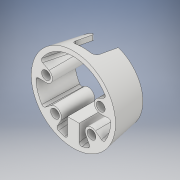
# Autodesk Inventor part: baseBottom
Saved by Autodesk Inventor 2018 (Build 220112000, 112)
## iProperties
Created: 2017-04-10
Part Number: baseBottom
Material: ABS Plastic
Document SubType Name: Modeling
Designer: dkt01
Density: 1.06 g/cm^3
Appearance: Smooth - White
Author: dkt01
Autodesk Inventor part; units mm, degrees
ref_plane "YZ Plane" through (0, 0, 0) normal (1, 0, 0) x (0, 1, 0)
ref_plane "XZ Plane" through (0, 0, 0) normal (0, 1, 0) x (-1, 0, 0)
sketch "Sketch1" plane through (0, 0, 0) normal (0, 0, 1) x (1, 0, 0)
  circle A0 centre (0, 0) radius 30.643
  circle A1 centre (0, 0) radius 26.581
  line L0 (0, 0) -> (0, 34.214349)
  line L1 (10, 28.965384) -> (10, 24.628227)
  line L2 (-24, 19.052387) -> (-24, 11.425829)
  dimension "d51" = 53.162
  dimension "d53" = 10
  dimension "d54" = 24
  dimension "d55" = 4.062
  constraints: 6 end point, 4 point on circle, 3 vertical, 2 centre point, 2 coincident
  measures "d51" diameter of A1
  measures "d53" distance between parallel lines of L0 L1
  measures "d54" distance between parallel lines of L2 L0
  measures "d55" radial gap between concentric circles of A0 A1
extrude "Extrusion1" add sketch "Sketch1" along normal blind 30 draft 10
shell "Shell1" thickness 4 removed faces 2 at (10.151889, -4.096582, 30) at (-7.737173, 3.588786, 0)
sketch "Sketch2" plane through (0, 0, 0) normal (0, 0, -1) x (-1, 0, 0)
  line L0 (0, 0) -> (0, 42.956518)
  line L1 (-10, 5.652174) -> (10, 5.652174)
  line L2 (10, 5.652174) -> (10, 52.710838)
  line L3 (10, 52.710838) -> (-10, 52.710838)
  line L4 (-10, 52.710838) -> (-10, 5.652174)
  dimension "d3" = 10
  dimension "d4" = 10
  constraints: 10 end point, 2 parallel, 1 horizontal, 1 perpendicular, 1 vertical
  measures "d3" distance between parallel lines of L0 L4
  measures "d4" distance between parallel lines of L2 L0
extrude "Extrusion2" cut sketch "Sketch2" against normal blind 22
ref_plane "Work Plane1" through (0, 0, 1.7) normal (0, 0, -1) x (-1, 0, 0)
sketch "Sketch3" plane through (0, 0, 1.7) normal (0, 0, -1) x (-1, 0, 0)
  arc A0 (-10, 24.628544) -> (10, 24.628544) centre (0, 0) ccw
  circle A1 centre (-23.304766, 6.454224) radius 2
  circle A2 centre (-15.445766, -18.129473) radius 2
  circle A3 centre (15.640493, -18.228751) radius 2
  circle A4 centre (23.319503, 6.396996) radius 2
  circle A5 centre (-23.304766, 6.454224) radius 3.75
  circle A6 centre (-15.445766, -18.129473) radius 3.75
  circle A7 centre (15.640493, -18.228751) radius 3.75
  circle A8 centre (23.319503, 6.396996) radius 3.75
  circle A9 centre (-23.304766, 6.454224) radius 5.5
  circle A10 centre (-15.445766, -18.129473) radius 5.5
  circle A11 centre (15.640493, -18.228751) radius 5.5
  circle A12 centre (23.319503, 6.396996) radius 5.5
  line L0 (-20.945766, 0) -> (17.819503, 0)
  line L1 (-23.304766, 6.454224) -> (0, 0)
  line L2 (0, 0) -> (23.319503, 6.396996)
  line L3 (15.640493, -18.228751) -> (0, 0)
  line L4 (0, 0) -> (-15.445766, -18.129473)
  dimension "d19" = 4
  dimension "d20" = 4
  dimension "d21" = 4
  dimension "d22" = 4
  dimension "d23" = 7.5
  dimension "d24" = 7.5
  dimension "d25" = 7.5
  dimension "d26" = 7.5
  dimension "d29" = 11
  dimension "d30" = 11
  dimension "d31" = 11
  dimension "d32" = 11
  dimension "d56" = 15.34
  dimension "d57" = 15.48
  dimension "d58" = 49.57
  dimension "d59" = 49.37
  dimension "d60" = 24.181
  dimension "d61" = 24.182
  dimension "d62" = 23.817
  dimension "d63" = 24.019
  constraints: 12 centre point, 12 coincident, 10 end point, 1 horizontal
  measures "d19" diameter of A1
  measures "d20" diameter of A2
  measures "d21" diameter of A3
  measures "d22" diameter of A4
  measures "d23" diameter of A5
  measures "d24" diameter of A6
  measures "d25" diameter of A7
  measures "d26" diameter of A8
  measures "d29" diameter of A9
  measures "d30" diameter of A10
  measures "d31" diameter of A12
  measures "d32" diameter of A11
  measures "d56" angle of L0 L2
  measures "d57" angle of L0 L1
  measures "d58" angle of L4 L0
  measures "d59" angle of L3 L0
  measures "d60" distance of L1.end L2.end
  measures "d61" distance of L1.start L1.end
  measures "d62" distance of L1.end L4.end
  measures "d63" distance of L3.start L1.end
sketch "Sketch4" plane through (0, 0, 30) normal (0, 0, 1) x (1, 0, 0)
  line L0 (5, -15) -> (-5, -15)
  line L1 (-5, -15) -> (-5, -35.527022)
  line L2 (-5, -35.527022) -> (5, -35.527022)
  line L3 (5, -35.527022) -> (5, -15)
  line L4 (0, 0) -> (0, -18.124685)
  dimension "d11" = 5
  dimension "d12" = 5
  dimension "d13" = 15
  constraints: 10 end point, 2 parallel, 1 horizontal, 1 perpendicular, 1 vertical
  measures "d11" distance between parallel lines of L4 L3
  measures "d12" distance between parallel lines of L1 L4
  measures "d13" distance from line of L4.start L0
extrude "Extrusion3" add sketch "Sketch4" against normal up to surface (28.3 mm away) from surface at 0
fillet "Fillet1" radius 2 2 edges at (-5, -28.8365, 15.2299) (5, -28.8365, 15.2299)
sketch "Sketch5" plane through (0, 0, 1.7) normal (0, 0, -1) x (-1, 0, 0)
  arc A0 (-5, -30.536112) -> (5, -30.536112) centre (0, 0) ccw
  line L0 (-5, -35.527022) -> (-5, -30.536112)
  line L1 (5, -35.527022) -> (-5, -35.527022)
  line L2 (5, -30.536112) -> (5, -35.527022)
extrude "Extrusion4" cut sketch "Sketch5" against normal up to surface round surface about axis through (0, 0, 0) along (0, 0, 1) radius 30.643 half angle 10 far side no
extrude "Extrusion5" cut sketch "Sketch3" against normal up to surface (30 mm away) from surface at 1.7 contours A5 A0 | A0 A5 | A6 A0 | A0 A6 | A8 A0 | A7 A0 | A0 A7 | A8 A0 | A1 | A2 | A3 | A4
ref_plane "Work Plane2" through (0, 0, 4.7) normal (0, 0, -1) x (-1, 0, 0)
sketch "Sketch6" plane through (0, 0, 4.7) normal (0, 0, -1) x (-1, 0, 0)
  circle A0 centre (15.640493, -18.228751) radius 3.75
  circle A1 centre (15.640493, -18.228751) radius 5.5
  circle A2 centre (23.319503, 6.396996) radius 3.75
  circle A3 centre (23.319503, 6.396996) radius 5.5
  circle A4 centre (-23.304766, 6.454224) radius 3.75
  circle A5 centre (-23.304766, 6.454224) radius 5.5
  circle A6 centre (-15.445766, -18.129473) radius 5.5
  circle A7 centre (-15.445766, -18.129473) radius 3.75
  point P0 (0, 0)
extrude "Extrusion6" add sketch "Sketch3" against normal up to surface (3 mm away) from surface at 0 contours A9 L1 A5 A0 | A0 A5 A9 | A5 A0 | A0 A5 | A0 A5 L1 A9 | A10 L4 A6 A0 | A0 A6 A10 | A6 A0 | A0 A6 | A10 A0 A6 L4 | L2 A8 A0 A12 | A12 A0 A8 L2 | L3 A7 A0 A11 | A11 A0 A7 L3 | A0 A7 A11 | A12 A0 A8 | A8 A0 | A7 A0 | A0 A7 | A8 A0
extrude "Extrusion7" add sketch "Sketch6" against normal up to surface (25.3 mm away) from surface at 0
sketch "Sketch7" plane through (0, 0, 30) normal (0, 0, 1) x (1, 0, 0)
  circle A0 centre (23.304766, 6.454224) radius 5.5
  circle A1 centre (15.445766, -18.129473) radius 5.5
  circle A2 centre (-15.640493, -18.228751) radius 5.5
  circle A3 centre (-23.319503, 6.396996) radius 5.5
  arc A4 (7.461091, -30.98547) -> (-7.461091, -30.98547) centre (0, 0) ccw
  line L0 (20.692585, 11.294318) -> (27.994029, 15.23488)
  line L1 (23.554687, 0.959905) -> (31.84305, 1.33692)
  line L2 (18.71712, -13.708133) -> (25.687646, -18.865631)
  line L3 (10.560918, -20.656972) -> (14.545682, -28.35825)
  line L4 (-10.769372, -20.782607) -> (-14.699521, -28.278814)
  line L5 (-18.904864, -13.802254) -> (-25.716836, -18.825821)
  line L6 (-23.555947, 0.902081) -> (-31.846234, 1.258809)
  line L7 (-20.719112, 11.243434) -> (-28.031028, 15.166695)
  constraints: 16 end point, 8 point on circle, 8 tangent, 9 other
extrude "Extrusion8" add sketch "Sketch7" against normal up to surface (28.3 mm away) contours A0 L0 A4 L1 | A1 L2 A4 L3 | A2 L4 A4 L5 | A3 L6 A4 L7
sketch "Sketch8" plane through (0, 0, 1.7) normal (0, 0, -1) x (-0.9637237, -0.266902, 0)
  arc A0 (29.471794, 9.426955) -> (22.294932, 21.456704) centre (0, 0) ccw
  line L0 (30.354991, 9.712967) -> (29.471794, 9.426955)
  arc A1 (30.354991, 9.712967) -> (22.966145, 22.098041) centre (0, 0) ccw
  line L1 (22.294932, 21.456704) -> (22.966145, 22.098041)
  arc A2 (21.079068, -22.652307) -> (28.94146, -10.947422) centre (0, 0) ccw
  line L2 (21.713948, -23.329631) -> (21.079068, -22.652307)
  arc A3 (21.713948, -23.329631) -> (29.808573, -11.279015) centre (0, 0) ccw
  line L3 (28.94146, -10.947422) -> (29.808573, -11.279015)
  arc A4 (-19.148683, -24.306009) -> (-6.258067, -30.303312) centre (0, 0) ccw
  line L4 (-19.720518, -25.037339) -> (-19.148683, -24.306009)
  arc A5 (-19.720518, -25.037339) -> (-6.449145, -31.211788) centre (0, 0) ccw
  line L5 (-6.258067, -30.303312) -> (-6.449145, -31.211788)
  arc A6 (-30.139717, 7.003683) -> (-30.139717, -7.003683) centre (0, 0) ccw
  line L6 (-31.044728, 7.210552) -> (-30.139717, 7.003683)
  arc A7 (-31.044728, 7.210552) -> (-31.044728, -7.210552) centre (0, 0) ccw
  line L7 (-30.139717, -7.003683) -> (-31.044728, -7.210552)
extrude "Extrusion9" cut sketch "Sketch8" against normal up to surface round surface about axis through (0, 0, 0) along (0, 0, 1) radius 30.643 half angle 10 far side no
fillet "Fillet2" radius 2 8 edges at (23.5966, -17.3185, 15.248) (13.3503, -26.048, 15.248) (29.2445, 1.2187, 15.248) (25.7049, 13.9995, 15.248) (-29.2474, 1.147, 15.248) (-25.7389, 13.9369, 15.248) (-13.4917, -25.975, 15.248) (-23.6233, -17.282, 15.248)
fillet "Fillet3" radius 4 2 edges at (10, 30.9072, 22) (-10, 30.9072, 22)
chamfer "Chamfer1" distance 1 angle 45 4 edges at (-21.3195, 6.397, 4.7) (-13.6405, -18.2288, 4.7) (17.4458, -18.1295, 4.7) (25.3048, 6.4542, 4.7)
split "Split1" plane through (0, 0, 1.7) removes the side toward (0, 0, -1)
fillet "Fillet5" radius 2 1 edges at (-10, 27.117, 1.7)
body "Solid1"
